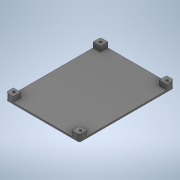
# Autodesk Inventor part: SensorsC_Holder
Saved by Autodesk Inventor 2020 (Build 240168000, 168)
## iProperties
Created: 2020-04-23
Part Number: SensorsC_Holder
Material: Типовые
Document SubType Name: Modeling
Designer: Михаил
Density: 1 g/cm^3
Appearance: По умолчанию
Author: Михаил
Autodesk Inventor part; units mm, degrees
ref_plane "YZ Plane" through (0, 0, 0) normal (1, 0, 0) x (0, 1, 0)
ref_plane "XZ Plane" through (0, 0, 0) normal (0, 1, 0) x (-1, 0, 0)
ref_plane "XY Plane" through (0, 0, 0) normal (0, 0, 1) x (1, 0, 0)
sketch "Эскиз1" plane through (0, 0, 0) normal (0, 1, 0) x (-1, 0, 0)
  line L0 (0, 0) -> (70, 0)
  line L1 (70, 0) -> (70, -90)
  line L2 (70, -90) -> (0, -90)
  line L3 (0, -90) -> (0, 0)
  dimension "d0" = 70
  dimension "d1" = 90
  constraints: 8 end point, 2 parallel, 1 horizontal, 1 perpendicular
  measures "d0" distance of L1.end L2.end
  measures "d1" distance of L0.end L1.end
extrude "Выдавливание1" add sketch "Эскиз1" along normal blind 1.5
sketch "Эскиз2" plane through (0, 1.5, 0) normal (0, 1, 0) x (1, 0, 0)
  line L0 (0, 0) -> (0, 90) projected
  line L1 (0, 0) -> (-7, 0)
  line L2 (-7, 0) -> (-7, 7)
  line L3 (-7, 7) -> (0, 7)
  line L4 (0, 7) -> (0, 0)
  line L5 (-70, 0) -> (0, 0) projected
  line L6 (-70, 0) -> (-63, 0)
  line L7 (-63, 0) -> (-63, 7)
  line L8 (-63, 7) -> (-70, 7)
  line L9 (-70, 7) -> (-70, 0)
  line L10 (0, 90) -> (-70, 90) projected
  line L11 (-70, 90) -> (-63, 90)
  line L12 (-63, 90) -> (-63, 83)
  line L13 (-63, 83) -> (-70, 83)
  line L14 (-70, 83) -> (-70, 90)
  line L15 (0, 90) -> (-7, 90)
  line L16 (-7, 90) -> (-7, 83)
  line L17 (-7, 83) -> (0, 83)
  line L18 (0, 83) -> (0, 90)
  point P0 (0, 7)
  point P1 (0, 83)
  point P2 (-63, 0)
  dimension "d4" = 7
  dimension "d5" = 7
  dimension "d6" = 7
  dimension "d7" = 7
  dimension "d8" = 7
  dimension "d9" = 7
  dimension "d10" = 7
  dimension "d11" = 7
  constraints: 32 end point, 8 parallel, 4 horizontal, 4 perpendicular
  measures "d4" distance of L2.end L3.end
  measures "d5" distance of L1.end L2.end
  measures "d6" distance of L8.end L7.end
  measures "d7" distance of L7.end L6.end
  measures "d8" distance of L12.end L13.end
  measures "d9" distance of L11.end L12.end
  measures "d10" distance of L17.end L16.end
  measures "d11" distance of L16.end L15.end
extrude "Выдавливание2" add sketch "Эскиз2" along normal blind 5
sketch "Эскиз3" plane through (0, 6.5, 0) normal (0, 1, 0) x (1, 0, 0)
  circle A0 centre (-2.75, 86.25) radius 1.25
  circle A1 centre (-66.25, 86.25) radius 1.25
  circle A2 centre (-66.25, 3.75) radius 1.25
  circle A3 centre (-2.75, 3.75) radius 1.25
  line L0 (-63, 90) -> (-70, 90) projected
  line L1 (0, 90) -> (-7, 90) projected
  line L2 (-70, 0) -> (-63, 0) projected
  line L3 (-7, 0) -> (0, 0) projected
  line L4 (-70, 90) -> (-70, 83) projected
  line L5 (0, 7) -> (0, 83) projected
  line L6 (-70, 7) -> (-70, 0) projected
  line L7 (0, 0) -> (0, 7) projected
  dimension "d14" = 2.5
  dimension "d15" = 2.5
  dimension "d16" = 2.5
  dimension "d17" = 2.5
  dimension "d18" = 3.75
  dimension "d19" = 3.75
  dimension "d20" = 3.75
  dimension "d21" = 3.75
  dimension "d22" = 3.75
  dimension "d23" = 2.75
  dimension "d24" = 3.75
  dimension "d25" = 2.75
  constraints: 4 centre point
  measures "d14" diameter of A0
  measures "d15" diameter of A1
  measures "d16" diameter of A2
  measures "d17" diameter of A3
  measures "d18" distance from line of L0 A1.centre
  measures "d19" distance from line of L1 A0.centre
  measures "d20" distance from line of L2 A2.centre
  measures "d21" distance from line of L3 A3.centre
  measures "d22" distance from line of L4 A1.centre
  measures "d23" distance from line of L5 A0.centre
  measures "d24" distance from line of L6 A2.centre
  measures "d25" distance from line of L7 A3.centre
extrude "Выдавливание3" cut sketch "Эскиз3" against normal blind 5
fillet "Сопряжение1" radius 2 4 edges at (0, 3.25, 0) (0, 3.25, -90) (-70, 3.25, -90) (-70, 3.25, 0)
